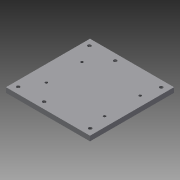
# Autodesk Inventor part: Motor Shim
Saved by Autodesk Inventor 2015 SP1 (Build 190203100, 203)
## iProperties
Created: 2016-03-22
Part Number: Motor Shim
Material: Generic
Document SubType Name: Modeling
Designer: Mac
Density: 1 g/cm^3
Appearance: Default
Author: Mac
Autodesk Inventor part; units mm, degrees
ref_plane "YZ Plane" through (0, 0, 0) normal (1, 0, 0) x (0, 1, 0)
ref_plane "XZ Plane" through (0, 0, 0) normal (0, 1, 0) x (-1, 0, 0)
ref_plane "XY Plane" through (0, 0, 0) normal (0, 0, 1) x (1, 0, 0)
sketch "Sketch2" plane through (0, 0, 0) normal (0, 1, 0) x (-1, 0, 0)
  line L0 (82.55, 82.55) -> (-82.55, 82.55)
  line L1 (-82.55, 82.55) -> (-82.55, -82.55)
  line L2 (-82.55, -82.55) -> (82.55, -82.55)
  line L3 (82.55, -82.55) -> (82.55, 82.55)
  point P0 (0, 0)
  point P1 (82.55, 0)
  point P2 (0, -82.55)
  dimension "d0" = 165.1
  dimension "d1" = 165.1
  constraints: 8 end point, 2 midpoint, 2 parallel, 1 horizontal, 1 horizontal alignment, 1 perpendicular, 1 vertical alignment
  measures "d0" distance of L2.end L0.start
  measures "d1" distance of L1.end L2.end
extrude "Extrusion1" add sketch "Sketch2" along normal blind 9.525
sketch "Sketch3" plane through (0, 9.525, 0) normal (0, 1, 0) x (1, 0, 0)
  line L0 (-82.55, 82.55) -> (-82.55, -82.55) projected
  line L1 (82.55, 82.55) -> (-82.55, 82.55) projected
  line L2 (115.57, 0) -> (-115.57, 0) projected
  point P0 (0, 0)
  point P1 (-71.12, 69.85)
  point P2 (-20.32, 69.85)
  point P3 (70.104, 69.85)
  point P4 (-71.12, -69.85)
  point P5 (-20.32, -69.85)
  point P6 (70.104, -69.85)
  dimension "d4" = 11.43
  dimension "d5" = 50.8
  dimension "d6" = 90.424
  dimension "d7" = 12.7
  constraints: 3 symmetric about line, 2 horizontal alignment
  measures "d4" distance from line of L0 point (-71.12, 69.85)
  measures "d5" distance of point (-20.32, 69.85) point (-71.12, 69.85)
  measures "d6" distance of point (70.104, 69.85) point (-20.32, 69.85)
  measures "d7" distance from line of L1 point (-71.12, 69.85)
hole "Hole1" at (-71.12, 9.525, -69.85) at (-20.32, 9.525, -69.85) at (70.104, 9.525, -69.85) at (-71.12, 9.525, 69.85) at (-20.32, 9.525, 69.85) at (70.104, 9.525, 69.85) direction (0, -1, 0) diameter 6.4008 end through all thread size "5/16-18 UNC" class "2B" standard "ANSI Unified Screw Threads"
sketch "Sketch4" plane through (0, 9.525, 0) normal (0, 1, 0) x (1, 0, 0)
  circle A0 centre (-20.32, -69.85) radius 3.2004 projected
  circle A1 centre (70.104, 69.85) radius 3.2004 projected
  circle A2 centre (-71.12, 69.85) radius 3.2004 projected
  circle A3 centre (-20.32, 69.85) radius 3.2004 projected
  circle A4 centre (-71.12, -69.85) radius 3.2004 projected
  circle A5 centre (70.104, -69.85) radius 3.2004 projected
  line L0 (-82.55, -82.55) -> (82.55, -82.55) projected
  line L1 (82.55, -82.55) -> (82.55, 82.55) projected
  line L2 (82.55, 82.55) -> (-82.55, 82.55) projected
  line L3 (-82.55, 82.55) -> (-82.55, -82.55) projected
  line L4 (-115.57, 0) -> (115.57, 0) projected
  point P0 (0, 0)
  point P1 (-50.7238, 35.0012)
  point P2 (63.5762, 35.0012)
  point P3 (-50.7238, -35.0012)
  point P4 (63.5762, -35.0012)
  dimension "d15" = 31.8262
  dimension "d16" = 114.3
  dimension "d17" = 47.5488
  constraints: 2 symmetric about line, 1 horizontal alignment
  measures "d15" distance from line of L3 point (-50.724, 35.001)
  measures "d16" distance of point (63.576, 35.001) point (-50.724, 35.001)
  measures "d17" distance from line of L2 point (-50.724, 35.001)
hole "Hole2" at (-50.7238, 9.525, -35.0012) at (63.5762, 9.525, -35.0012) at (-50.7238, 9.525, 35.0012) at (63.5762, 9.525, 35.0012) direction (0, -1, 0) diameter 4.9784 end through all thread size "1/4-20 UNC" class "2B" standard "ANSI Unified Screw Threads"
body "Solid1"
